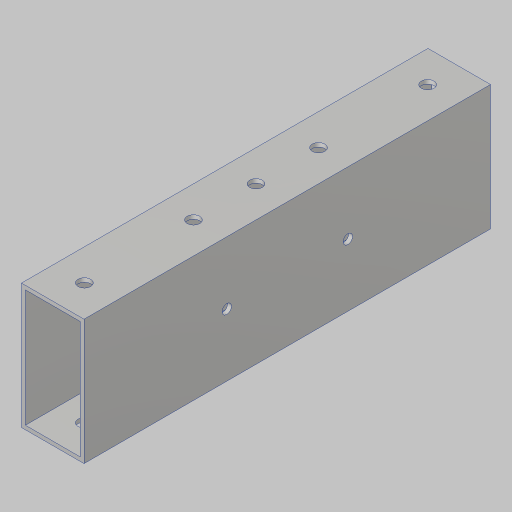
# Autodesk Inventor part: EL2-C-001
Saved by Autodesk Inventor 2023.5 (Build 275446000, 446)
## iProperties
RuleStatus: InUse
Created: 2025-01-11
Part Number: EL2-C-001
Material: Aluminum 6061
Document SubType Name: Modeling
Designer: brand
Mass: 304.185 g
Surface Area: 718.547 cm^2
Volume: 112.661 cm^3
Density: 2.7 g/cm^3
Appearance: Aluminum - Flat
AfterDocNew0: SHOW
AfterDocOpen0: SHOW
Author: brand
Autodesk Inventor part; units mm, degrees
ref_plane "YZ Plane" through (0, 0, 0) normal (1, 0, 0) x (0, 1, 0)
ref_plane "XZ Plane" through (0, 0, 0) normal (0, 1, 0) x (-1, 0, 0)
ref_plane "XY Plane" through (0, 0, 0) normal (0, 0, 1) x (1, 0, 0)
sketch "Sketch1" plane through (0, 0, 0) normal (0, 0, 1) x (1, 0, 0)
  line L0 (-12.7, -25.4) -> (12.7, -25.4)
  line L1 (12.7, -25.4) -> (12.7, 25.4)
  line L2 (12.7, 25.4) -> (-12.7, 25.4)
  line L3 (-12.7, 25.4) -> (-12.7, -25.4)
  line L4 (-12.7, -25.4) -> (12.7, 25.4) construction
  line L5 (12.7, -25.4) -> (-12.7, 25.4) construction
  line L6 (-11.1125, 23.8125) -> (11.1125, 23.8125)
  line L7 (11.1125, 23.8125) -> (11.1125, -23.8125)
  line L8 (11.1125, -23.8125) -> (-11.1125, -23.8125)
  line L9 (-11.1125, -23.8125) -> (-11.1125, 23.8125)
  point P0 (0, 0)
  dimension "width" = 25.4
  dimension "height" = 50.8
  dimension "thickness" = 1.5875
  constraints: 20 end point, 4 parallel, 2 midpoint, 2 perpendicular, 1 horizontal, 3 other
  measures "width" distance of L2.end L1.end
  measures "height" distance of L1.end L0.end
  measures "thickness" distance between parallel lines of L2 L6
extrude "Extrusion1" add sketch "Sketch1" along normal mid plane 165.1
sketch "Sketch5" plane through (-12.7, 25.4, 82.55) normal (0, 1, 0) x (1, 0, 0)
  point P0 (12.7, 82.55)
  point P1 (12.7, 82.55)
  point P2 (12.7, 107.95)
  point P3 (12.7, 57.15)
  dimension "d28" = 25.4
  dimension "d29" = 25.4
  constraints: 2 vertical alignment, 1 coincident
  measures "d28" distance of point (12.7, 82.55) point (12.7, 107.95)
  measures "d29" distance of point (12.7, 57.15) point (12.7, 82.55)
hole "Hole3" at (0, 25.4, 0) at (0, 25.4, -25.4) at (0, 25.4, 25.4) direction (0, -1, 0) diameter 5.1054 end through all clearance for "Flat Head Machine Screw (82)" size "#10" standard "Ansi Unified Screw Threads"
sketch "Sketch6" plane through (-12.7, 25.4, 82.55) normal (0, 1, 0) x (1, 0, 0)
  line L0 (12.7, 152.273) -> (12.7, 12.827) construction
  line L1 (0, 165.1) -> (25.4, 165.1) construction
  point P0 (12.7, 82.55)
  point P1 (12.7, 82.55)
  point P2 (12.7, 165.1)
  dimension "d37" = 139.446
  constraints: 2 end point, 2 midpoint, 1 coincident, 1 vertical, 1 vertical alignment
  measures "d37" distance of L0.start L0.end
hole "Hole4" at (0, 25.4, -69.723) at (0, 25.4, 69.723) direction (0, -1, 0) diameter 5.1054 end through all clearance for "Flat Head Machine Screw (82)" size "#10" standard "Ansi Unified Screw Threads"
sketch "Sketch7" plane through (12.7, -25.4, 82.55) normal (1, 0, 0) x (0, 0, -1)
  line L0 (57.9558, 25.4) -> (107.1442, 25.4) construction
  point P0 (82.55, 25.4)
  point P1 (82.55, 25.4)
  dimension "d45" = 49.1884
  constraints: 2 end point, 2 horizontal alignment, 1 coincident, 1 horizontal, 1 midpoint
  measures "d45" distance of L0.start L0.end
hole "Hole5" at (12.7, 0, 24.5942) at (12.7, 0, -24.5942) direction (-1, 0, 0) diameter 3.81 end through all clearance for "Flat Head Machine Screw (82)" size "#6" standard "Ansi Unified Screw Threads"
equation "\"d29\" = d28"
body "Solid1"
